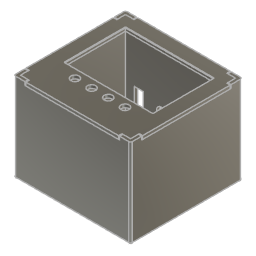
schnorriMat V1 (Autodesk Fusion 360 design; units mm, degrees)
Autodesk Fusion 360 part; units mm, degrees
sketch "Sketch2" plane through (0, 0, 0) normal (0, 0, 1) x (1, 0, 0)
  line L0 (-55, 60) -> (55, 60)
  line L1 (55, 60) -> (55, -60)
  line L2 (55, -60) -> (-55, -60)
  line L3 (-55, -60) -> (-55, 60)
  line L4 (0, 60) -> (0, -60) construction
  line L5 (55, 0) -> (-55, 0) construction
  line L6 (-55, 17.8) -> (55, 17.8) construction
  line L7 (-39.5, 45) -> (39.5, 45)
  line L8 (39.5, 45) -> (39.5, -9.4)
  line L9 (39.5, -9.4) -> (-39.5, -9.4)
  line L10 (-39.5, -9.4) -> (-39.5, 45)
  line L11 (39.5, 17.8) -> (-39.5, 17.8) construction
  line L12 (0, 45) -> (0, -9.4) construction
  line L13 (-55, -32) -> (55, -32) construction
  circle A0 centre (22.5, -32) radius 12.5
  circle A1 centre (-22.5, -32) radius 6.25
  line L14 (-6.3, -15.8) -> (-38.7, -15.8)
  line L15 (-38.7, -15.8) -> (-38.7, -48.2)
  line L16 (-38.7, -48.2) -> (-6.3, -48.2)
  line L17 (-6.3, -48.2) -> (-6.3, -15.8)
  line L18 (-6.3, -15.8) -> (-38.7, -48.2) construction
  line L19 (-38.7, -15.8) -> (-6.3, -48.2) construction
  line L20 (-4.3, -13.8) -> (-40.7, -13.8)
  line L21 (-40.7, -13.8) -> (-40.7, -50.2)
  line L22 (-40.7, -50.2) -> (-4.3, -50.2)
  line L23 (-4.3, -50.2) -> (-4.3, -13.8)
  line L24 (-32.5, -48.2) -> (-32.5, -50.2)
  line L25 (-38.7, -42) -> (-40.7, -42)
  line L26 (-22.5, -32) -> (-22.5, -50.2) construction
  point P0 (0, 17.8)
  point P1 (-22.5, -32)
  dimension "d1" = 110
  dimension "d6" = 120
  dimension "d7" = 79
  dimension "d8" = 54.4
  dimension "d9" = 15
  dimension "d12" = 25
  dimension "d13" = 12.5
  dimension "d15" = 32.4
  dimension "d16" = 32.4
  dimension "d17" = 45
  dimension "d18" = 22.5
  dimension "d19" = 28
  dimension "d42" = 2
  dimension "d63" = 10
  dimension "d64" = 10
  constraint horizontal L0
  constraint vertical L1
  constraint horizontal L2
  constraint vertical L3
  constraint midpoint L0 L4.start
  constraint midpoint L2 L4.end
  constraint midpoint L1 L5.start
  constraint midpoint L3 L5.end
  constraint midpoint L4 origin
  constraint coincident L3 L6.start
  constraint coincident L1 L6.end
  constraint perpendicular L1 L6
  constraint horizontal L7
  constraint vertical L8
  constraint horizontal L9
  constraint vertical L10
  constraint midpoint L8 L11.start
  constraint midpoint L10 L11.end
  constraint midpoint L7 L12.start
  constraint midpoint L9 L12.end
  constraint midpoint L11 P0
  constraint coincident L4 P0
  constraint collinear L6 L11
  constraint coincident L3 L13.start
  constraint coincident L1 L13.end
  constraint perpendicular L1 L13
  constraint coincident L13 A0.centre
  constraint coincident L13 P1
  constraint horizontal L14
  constraint perpendicular L14 L15
  constraint parallel L14 L16
  constraint parallel L15 L17
  constraint coincident L18 P1
  constraint coincident L19 P1
  constraint coincident P1 A1.centre
  constraint coincident L16 L24.start
  constraint perpendicular L16 L24
  constraint coincident L22 L24.end
  constraint coincident L15 L25.start
  constraint coincident L21 L25.end
  constraint perpendicular L21 L25
  constraint midpoint L22 L26.end
  measures "d1" distance of L0.start L0.end
  measures "d6" distance of L0.start L2.end
  measures "d7" distance of L7.start L7.end
  measures "d8" distance of L7.end L8.end
  measures "d9" distance of L0 L7
  measures "d12" diameter of A0
  measures "d13" diameter of A1
  measures "d15" distance of L15.end L16.end
  measures "d16" distance of L14.end L15.end
  measures "d17" distance of A0.centre P1
  measures "d18" distance of L4 P1
  measures "d19" distance of L2 L13
  measures "d63" distance of L13 L25
  measures "d64" distance of L24 L26
sketch "Sketch3" plane through (0, 0, 0) normal (0, 0, 1) x (1, 0, 0)
  line L0 (-55, 60) -> (55, 60)
  line L1 (55, 60) -> (55, -60)
  line L2 (55, -60) -> (-55, -60)
  line L3 (-55, -60) -> (-55, 60)
  line L4 (55, 0) -> (-55, 0) construction
  line L5 (0, 60) -> (0, -60) construction
  line L6 (-52.6, 57.6) -> (52.6, 57.6)
  line L7 (52.6, 57.6) -> (52.6, -57.6)
  line L8 (52.6, -57.6) -> (-52.6, -57.6)
  line L9 (-52.6, -57.6) -> (-52.6, 57.6)
  line L10 (-39.6, 57.6) -> (-39.6, 44.6)
  line L11 (-39.6, 44.6) -> (-52.6, 44.6)
  line L12 (-39.6, 51.1) -> (-52.6, 51.1) construction
  line L13 (-46.1, 44.6) -> (-46.1, 57.6) construction
  circle A0 centre (-46.1, 51.1) radius 5
  line L14 (-40.4, 57.6) -> (-40.4, 60)
  line L15 (-52.6, 45.4) -> (-55, 45.4)
  line L16 (-52.6, 44.6) -> (-55, 44.6)
  line L17 (-39.6, 57.6) -> (-39.6, 60)
  line L18 (39.6, 57.6) -> (39.6, 60)
  line L19 (40.4, 57.6) -> (40.4, 60)
  circle A1 centre (46.1, 51.1) radius 5
  line L20 (39.6, 57.6) -> (39.6, 44.6)
  line L21 (39.6, 44.6) -> (52.6, 44.6)
  line L22 (52.6, 44.6) -> (55, 44.6)
  line L23 (52.6, 45.4) -> (55, 45.4)
  line L24 (40.4, -57.6) -> (40.4, -60)
  line L25 (39.6, -57.6) -> (39.6, -60)
  line L26 (39.6, -57.6) -> (39.6, -44.6)
  circle A2 centre (46.1, -51.1) radius 5
  line L27 (39.6, -44.6) -> (52.6, -44.6)
  line L28 (52.6, -44.6) -> (55, -44.6)
  line L29 (52.6, -45.4) -> (55, -45.4)
  line L30 (-39.6, -57.6) -> (-39.6, -44.6)
  line L31 (-39.6, -57.6) -> (-39.6, -60)
  line L32 (-40.4, -57.6) -> (-40.4, -60)
  circle A3 centre (-46.1, -51.1) radius 5
  line L33 (-39.6, -44.6) -> (-52.6, -44.6)
  line L34 (-52.6, -44.6) -> (-55, -44.6)
  line L35 (-52.6, -45.4) -> (-55, -45.4)
  dimension "d20" = 110
  dimension "d21" = 120
  dimension "d22" = 2.4
  dimension "d23" = 13
  dimension "d26" = 10
  dimension "d27" = 0.8
  dimension "d28" = 0.8
  constraint horizontal L0
  constraint vertical L1
  constraint horizontal L2
  constraint vertical L3
  constraint midpoint L1 L4.start
  constraint midpoint L3 L4.end
  constraint midpoint L0 L5.start
  constraint midpoint L2 L5.end
  constraint midpoint L4 origin
  constraint coincident L6 L10.start
  constraint perpendicular L6 L10
  constraint coincident L9 L11.end
  constraint perpendicular L9 L11
  constraint midpoint L10 L12.start
  constraint coincident L9 L12.end
  constraint perpendicular L9 L12
  constraint midpoint L11 L13.start
  constraint coincident L6 L13.end
  constraint perpendicular L6 L13
  constraint midpoint L12 A0.centre
  constraint equal L10 L11
  constraint coincident L6 L14.start
  constraint coincident L0 L14.end
  constraint perpendicular L0 L14
  constraint coincident L9 L15.start
  constraint coincident L3 L15.end
  constraint perpendicular L3 L15
  constraint coincident L3 L16.end
  constraint perpendicular L3 L16
  constraint coincident L0 L17.end
  constraint perpendicular L0 L17
  constraint symmetric L5 L10.start L18.start
  constraint symmetric L5 L10.end L20.end
  constraint symmetric L5 L11.end L21.end
  constraint symmetric L5 A0 A1
  constraint symmetric L5 L14.start L19.start
  constraint symmetric L5 L14.end L19.end
  constraint symmetric L5 L15.start L23.start
  constraint symmetric L5 L15.end L23.end
  constraint symmetric L5 L16.end L22.end
  constraint symmetric L5 L17.end L18.end
  constraint symmetric L4 L10.start L30.start
  constraint symmetric L4 L10.end L30.end
  constraint symmetric L4 L11.end L33.end
  constraint symmetric L4 A0 A3
  constraint symmetric L4 L14.start L32.start
  constraint symmetric L4 L14.end L32.end
  constraint symmetric L4 L15.start L35.start
  constraint symmetric L4 L15.end L35.end
  constraint symmetric L4 L16.end L34.end
  constraint symmetric L4 L17.end L31.end
  constraint symmetric L4 L18.start L25.start
  constraint symmetric L4 L18.end L25.end
  constraint symmetric L4 L19.start L24.start
  constraint symmetric L4 L19.end L24.end
  constraint symmetric L4 A1 A2
  constraint symmetric L4 L20.end L26.end
  constraint symmetric L4 L21.end L27.end
  constraint symmetric L4 L22.end L28.end
  constraint symmetric L4 L23.start L29.start
  constraint symmetric L4 L23.end L29.end
  measures "d20" distance of L0.start L0.end
  measures "d21" distance of L0.start L2.end
  measures "d23" distance of L10.start L10.end
  measures "d26" diameter of A0
  measures "d27" distance of L14 L17
  measures "d28" distance of L15 L16
extrude "Extrude1" add sketch "Sketch3" along normal blind 2 contours L0 L3 L6 L9 L14 L15 | L0 L6 L14 L17 | L3 L9 L15 L16 | L0 L6 L17 L18 | L6 L9 L10 L11 | L3 L9 L16 L34 | L0 L6 L18 L19 | L6 L7 L8 L9 L10 L11 L20 L21 L26 L27 L30 L33 | L3 L9 L34 L35 | L0 L1 L6 L7 L19 L23 | L6 L7 L20 L21 | L2 L3 L8 L9 L32 L35 | L8 L9 L30 L33 | L1 L7 L22 L23 | L1 L7 L22 L28 | L2 L8 L31 L32 | L2 L8 L25 L31 | L1 L7 L28 L29 | L7 L8 L26 L27 | L2 L8 L24 L25 | L1 L2 L7 L8 L24 L29 | A0 | A1 | A2 | A3 makes body 1
extrude "Extrude2" add sketch "Sketch3" along normal blind 77 contours L0 L3 L6 L9 L14 L15 | L0 L6 L14 L17 | L3 L9 L15 L16 | L0 L6 L17 L18 | L3 L9 L16 L34 | L0 L6 L18 L19 | L3 L9 L34 L35 | L0 L1 L6 L7 L19 L23 | L2 L3 L8 L9 L32 L35 | L1 L7 L22 L23 | L1 L7 L22 L28 | L2 L8 L31 L32 | L2 L8 L25 L31 | L1 L7 L28 L29 | L2 L8 L24 L25 | L1 L2 L7 L8 L24 L29 bodies 1
extrude "Extrude3" add sketch "Sketch3" along normal blind 3 from surface at 77 contours L0 L3 L6 L9 L14 L15 | L0 L1 L6 L7 L19 L23 | L2 L3 L8 L9 L32 L35 | L1 L2 L7 L8 L24 L29 bodies 1
extrude "Extrude4" add sketch "Sketch2" along normal blind 3 from surface at 77 separate body contours L0 L1 L2 L3 | L14 L15 L16 L17 | L14 L15 L16 L17 L20 L21 L22 L23 L24 L25 | L15 L16 L21 L22 L24 L25 makes body 2
extrude "Extrude5" cut sketch "Sketch3" along normal through all contours L0 L3 L6 L9 L14 L15 | L0 L6 L14 L17 | L3 L9 L15 L16 | L0 L6 L18 L19 | L3 L9 L34 L35 | L0 L1 L6 L7 L19 L23 | L2 L3 L8 L9 L32 L35 | L1 L7 L22 L23 | L2 L8 L31 L32 | L1 L7 L28 L29 | L2 L8 L24 L25 | L1 L2 L7 L8 L24 L29 bodies 2
extrude "Extrude6" add sketch "Sketch3" along normal up to surface (75 mm away) from surface at 2 contours L6 L9 L10 L11 | L6 L7 L20 L21 | L8 L9 L30 L33 | L7 L8 L26 L27 | A0 | A1 | A2 | A3 bodies 1
extrude "Extrude7" cut sketch "Sketch3" against normal blind 1.5 from surface at 77 contours A0 | A1 | A2 | A3 bodies 1
fillet "Fillet1" radius 0.4 4 edges at (-52.6, 57.6, 78.5) (52.6, 57.6, 78.5) (52.6, -57.6, 78.5) (-52.6, -57.6, 78.5) on bodies 2
extrude "Extrude8" add sketch "Sketch2" against normal blind 5 from surface at 77 contours L14 L15 L16 L17 L20 L21 L22 L23 L24 L25 bodies 2
extrude "Extrude9" cut sketch "Sketch3" along normal blind 1.5 from surface at 77 contours A0 | A1 | A2 | A3 bodies 2
fillet "Fillet2" radius 5 4 edges at (-39.6, -44.6, 39.5) (-39.6, 44.6, 39.5) (39.6, 44.6, 39.5) (39.6, -44.6, 39.5) on bodies 1
fillet "Fillet4" radius 2.5 8 edges at (39.6, 57.6, 39.5) (52.6, 44.6, 39.5) (52.6, -44.6, 39.5) (39.6, -57.6, 39.5) (-39.6, -57.6, 39.5) (-52.6, -44.6, 39.5) (-52.6, 44.6, 39.5) (-39.6, 57.6, 39.5) on bodies 1
fillet "Fillet5" radius 1.2 4 edges at (55, 60, 40) (-55, 60, 40) (-55, -60, 40) (55, -60, 40) on bodies 1
sketch "Sketch5" plane through (0, 0, 0) normal (0, 1, 0) x (1, 0, 0)
  line L0 (-55, 0) -> (55, 0)
  line L1 (55, 0) -> (55, -80)
  line L2 (55, -80) -> (-55, -80)
  line L3 (-55, -80) -> (-55, 0)
  line L4 (55, -20) -> (-55, -20) construction
  circle A0 centre (-35, -20) radius 4
  line L5 (-19, -28) -> (-11, -28)
  line L6 (-11, -28) -> (-11, -12)
  line L7 (-11, -12) -> (-19, -12)
  line L8 (-19, -12) -> (-19, -28)
  line L9 (-19, -20) -> (-11, -20) construction
  line L10 (-15, -28) -> (-15, -12) construction
  dimension "d69" = 80
  dimension "d70" = 110
  dimension "d71" = 8
  dimension "d72" = 8
  dimension "d73" = 16
  dimension "d74" = 20
  dimension "d75" = 20
  dimension "d76" = 20
  constraint horizontal L0
  constraint vertical L1
  constraint horizontal L2
  constraint vertical L3
  constraint midpoint L0 origin
  constraint coincident L1 L4.start
  constraint coincident L3 L4.end
  constraint perpendicular L3 L4
  constraint coincident L4 A0.centre
  constraint horizontal L5
  constraint vertical L6
  constraint horizontal L7
  constraint vertical L8
  constraint midpoint L8 L9.start
  constraint midpoint L6 L9.end
  constraint midpoint L5 L10.start
  constraint midpoint L7 L10.end
  constraint collinear L4 L9
  measures "d69" distance of L0.start L2.end
  measures "d70" distance of L0.start L0.end
  measures "d71" diameter of A0
  measures "d72" distance of L5.start L5.end
  measures "d73" distance of L5.start L7.end
  measures "d74" distance of A0.centre L10
  measures "d75" distance of L0 L4
  measures "d76" distance of L3 A0.centre
extrude "Extrude10" cut sketch "Sketch5" along normal blind 85 contours A0 | L5 L6 L7 L8 bodies 1
sketch "Sketch1" plane through (0, 0, 0) normal (0, 0, 1) x (1, 0, 0) in component "V2"
  line L0 (39.5, 27.2) -> (-39.5, 27.2)
  line L1 (-39.5, 27.2) -> (-39.5, -27.2)
  line L2 (-39.5, -27.2) -> (39.5, -27.2)
  line L3 (39.5, -27.2) -> (39.5, 27.2)
  line L4 (39.5, 27.2) -> (-39.5, -27.2) construction
  line L5 (-39.5, 27.2) -> (39.5, -27.2) construction
  line L6 (-49.5, 37.2) -> (49.5, 37.2)
  line L7 (49.5, 37.2) -> (49.5, -57.2)
  line L8 (49.5, -57.2) -> (-49.5, -57.2)
  line L9 (-49.5, -57.2) -> (-49.5, 37.2)
  line L10 (0, 37.2) -> (0, -57.2) construction
  line L11 (-49.5, -35.2) -> (49.5, -35.2) construction
  circle A0 centre (-7.5, -35.2) radius 3.7
  circle A1 centre (-22.5, -35.2) radius 3.7
  circle A2 centre (22.5, -35.2) radius 3.7
  circle A3 centre (7.5, -35.2) radius 3.7
  line L12 (52.5, 40.2) -> (52.5, -60.2)
  line L13 (52.5, -60.2) -> (-52.5, -60.2)
  line L14 (-52.5, -60.2) -> (-52.5, 40.2)
  line L15 (-52.5, 40.2) -> (52.5, 40.2)
  dimension "d79" = 79
  dimension "d80" = 54.4
  dimension "d81" = 10
  dimension "d82" = 10
  dimension "d83" = 30
  dimension "d85" = 7.4
  dimension "d86" = 15
  dimension "d87" = 7.5
  dimension "d88" = -3
  dimension "d109" = 8
  constraint horizontal L0
  constraint perpendicular L0 L1
  constraint parallel L0 L2
  constraint parallel L1 L3
  constraint coincident L4 origin
  constraint coincident L5 origin
  constraint horizontal L6
  constraint vertical L7
  constraint horizontal L8
  constraint vertical L9
  constraint midpoint L6 L10.start
  constraint midpoint L8 L10.end
  constraint coincident origin L10
  constraint coincident L9 L11.start
  constraint coincident L7 L11.end
  constraint perpendicular L7 L11
  constraint coincident L11 A0.centre
  constraint coincident L11 A1.centre
  constraint equal A0 A1
  constraint symmetric L10 A0 A3
  constraint symmetric L10 A1 A2
  measures "d79" distance of L1.end L2.end
  measures "d80" distance of L0.end L1.end
  measures "d81" distance of L0 L6
  measures "d82" distance of L1 L9
  measures "d83" distance of L2 L8
  measures "d85" diameter of A0
  measures "d86" distance of A0.centre A1.centre
  measures "d87" distance of L10 A0.centre
  measures "d109" distance of L2 L11
sketch "Sketch2 (2)" plane through (0, 0, 0) normal (0, 0, 1) x (1, 0, 0) in component "V2"
  line L0 (-49.5, 37.2) -> (49.5, 37.2)
  line L1 (49.5, 37.2) -> (49.5, -57.2)
  line L2 (49.5, -57.2) -> (-49.5, -57.2)
  line L3 (-49.5, -57.2) -> (-49.5, 37.2)
  line L4 (-52.5, 40.2) -> (52.5, 40.2)
  line L5 (52.5, 40.2) -> (52.5, -60.2)
  line L6 (52.5, -60.2) -> (-52.5, -60.2)
  line L7 (-52.5, -60.2) -> (-52.5, 40.2)
  line L8 (0, 40.2) -> (0, -60.2) construction
  line L9 (52.5, -10) -> (-52.5, -10) construction
  line L10 (-42.5, 40.2) -> (-42.5, 37.2)
  line L11 (-41.7, 40.2) -> (-41.7, 37.2)
  line L12 (-49.5, 30.2) -> (-52.5, 30.2)
  line L13 (-52.5, 29.4) -> (-49.5, 29.4)
  line L14 (41.7, 40.2) -> (41.7, 37.2)
  line L15 (42.5, 40.2) -> (42.5, 37.2)
  line L16 (49.5, 30.2) -> (52.5, 30.2)
  line L17 (52.5, 29.4) -> (49.5, 29.4)
  line L18 (-41.7, -60.2) -> (-41.7, -57.2)
  line L19 (-42.5, -60.2) -> (-42.5, -57.2)
  line L20 (-49.5, -50.2) -> (-52.5, -50.2)
  line L21 (-52.5, -49.4) -> (-49.5, -49.4)
  line L22 (42.5, -60.2) -> (42.5, -57.2)
  line L23 (41.7, -60.2) -> (41.7, -57.2)
  line L24 (49.5, -50.2) -> (52.5, -50.2)
  line L25 (52.5, -49.4) -> (49.5, -49.4)
  point P0 (-49.5, 37.2)
  point P1 (49.5, -57.2)
  dimension "d89" = -3
  dimension "d90" = 0.8
  dimension "d91" = 0.8
  dimension "d92" = 10
  dimension "d93" = 10
  constraint horizontal L0
  constraint vertical L1
  constraint horizontal L2
  constraint vertical L3
  constraint coincident P0 L0.start
  constraint coincident P1 L1.end
  constraint midpoint L4 L8.start
  constraint midpoint L6 L8.end
  constraint midpoint L5 L9.start
  constraint midpoint L7 L9.end
  constraint coincident L4 L10.start
  constraint coincident L0 L10.end
  constraint perpendicular L0 L10
  constraint coincident L4 L11.start
  constraint coincident L0 L11.end
  constraint perpendicular L0 L11
  constraint coincident L3 L12.start
  constraint coincident L7 L12.end
  constraint perpendicular L7 L12
  constraint coincident L7 L13.start
  constraint coincident L3 L13.end
  constraint perpendicular L3 L13
  constraint symmetric L8 L10.start L15.start
  constraint symmetric L8 L10.end L15.end
  constraint symmetric L8 L11.start L14.start
  constraint symmetric L8 L11.end L14.end
  constraint symmetric L8 L12.start L16.start
  constraint symmetric L8 L12.end L16.end
  constraint symmetric L8 L13.start L17.start
  constraint symmetric L8 L13.end L17.end
  constraint symmetric L9 L10.start L19.start
  constraint symmetric L9 L10.end L19.end
  constraint symmetric L9 L11.start L18.start
  constraint symmetric L9 L11.end L18.end
  constraint symmetric L9 L12.start L20.start
  constraint symmetric L9 L12.end L20.end
  constraint symmetric L9 L13.start L21.start
  constraint symmetric L9 L13.end L21.end
  constraint symmetric L9 L14.start L23.start
  constraint symmetric L9 L14.end L23.end
  constraint symmetric L9 L15.start L22.start
  constraint symmetric L9 L15.end L22.end
  constraint symmetric L9 L16.start L24.start
  constraint symmetric L9 L16.end L24.end
  constraint symmetric L9 L17.start L25.start
  constraint symmetric L9 L17.end L25.end
  measures "d90" distance of L10 L11
  measures "d91" distance of L12 L13
  measures "d92" distance of L7 L10
  measures "d93" distance of L4 L12
extrude "Extrude2'" add sketch "Sketch2 (2)" along normal blind 2 separate body makes body 3 in component "V2"
extrude "Extrude3'" add sketch "Sketch2 (2)" along normal blind 77 contours L0 L3 L4 L7 L10 L12 | L0 L4 L10 L11 | L3 L7 L12 L13 | L0 L4 L11 L14 | L3 L7 L13 L21 | L0 L4 L14 L15 | L3 L7 L20 L21 | L0 L1 L4 L5 L15 L16 | L2 L3 L6 L7 L19 L20 | L1 L5 L16 L17 | L2 L6 L18 L19 | L1 L5 L17 L25 | L2 L6 L18 L23 | L1 L5 L24 L25 | L2 L6 L22 L23 | L1 L2 L5 L6 L22 L24 bodies 3 in component "V2"
extrude "Extrude4'" add sketch "Sketch2 (2)" along normal blind 3 from surface at 77 contours L0 L3 L4 L7 L10 L12 | L0 L1 L4 L5 L15 L16 | L2 L3 L6 L7 L19 L20 | L1 L2 L5 L6 L22 L24 bodies 3 in component "V2"
extrude "Extrude5'" add sketch "Sketch1" along normal blind 3 from surface at 77 separate body contours L6 L7 L8 L9 makes body 4 in component "V2"
extrude "Extrude6'" add sketch "Sketch2 (2)" along normal up to surface (3 mm away) from surface at 77 contours L0 L4 L11 L14 | L3 L7 L13 L21 | L1 L5 L17 L25 | L2 L6 L18 L23 bodies 4 in component "V2"
fillet "Fillet1'" radius 1.6 4 edges at (-52.5, -60.2, 40) (52.5, -60.2, 40) (52.5, 40.2, 40) (-52.5, 40.2, 40) on bodies 3 in component "V2"
fillet "Fillet2'" radius 1.4 8 edges at (52.0314, 39.7314, 0) (52.5, -10, 0) (52.0314, -59.7314, 0) (0, -60.2, 0) (-52.0314, -59.7314, 0) (-52.5, -10, 0) (-52.0314, 39.7314, 0) (0, 40.2, 0) on bodies 3 in component "V2"
fillet "Fillet3" radius 0.4 4 edges at (0, 27.2, 80) (39.5, 0, 80) (-39.5, 0, 80) (0, -27.2, 80) on bodies 4 in component "V2"
sketch "Sketch3 (2)" plane through (0, 0, 0) normal (0, 1, 0) x (1, 0, 0) in component "V2"
  line L0 (52.5, 0) -> (-52.5, 0)
  line L1 (-52.5, 0) -> (-52.5, -77)
  line L2 (-52.5, -77) -> (52.5, -77)
  line L3 (52.5, -77) -> (52.5, 0)
  line L4 (0, -77) -> (0, 0) construction
  line L5 (-52.5, -20) -> (52.5, -20) construction
  line L6 (-33.5, -28) -> (-41.5, -28)
  line L7 (-41.5, -28) -> (-41.5, -12)
  line L8 (-41.5, -12) -> (-33.5, -12)
  line L9 (-33.5, -12) -> (-33.5, -28)
  line L10 (-33.5, -20) -> (-41.5, -20) construction
  circle A0 centre (-17.5, -20) radius 4
  line L11 (-37.5, -28) -> (-37.5, -12) construction
  point P0 (52.5, 0)
  point P1 (-37.5, -20)
  dimension "d118" = 8
  dimension "d119" = 16
  dimension "d120" = 8
  dimension "d121" = 20
  dimension "d122" = 15
  dimension "d123" = 20
  constraint horizontal L0
  constraint vertical L1
  constraint horizontal L2
  constraint vertical L3
  constraint midpoint L2 L4.start
  constraint midpoint L0 L4.end
  constraint coincident L4.end origin
  constraint coincident P0 L0.start
  constraint coincident L1 L5.start
  constraint coincident L3 L5.end
  constraint perpendicular L3 L5
  constraint horizontal L6
  constraint vertical L7
  constraint horizontal L8
  constraint vertical L9
  constraint midpoint L9 L10.start
  constraint midpoint L7 L10.end
  constraint coincident L5 A0.centre
  constraint midpoint L6 L11.start
  constraint midpoint L8 L11.end
  constraint midpoint L11 P1
  constraint coincident L5 P1
  measures "d118" distance of L6.start L6.end
  measures "d119" distance of L6.start L8.end
  measures "d120" diameter of A0
  measures "d121" distance of L0 L5
  measures "d122" distance of L1 L11
  measures "d123" distance of A0.centre L11
extrude "Extrude7'" cut sketch "Sketch3 (2)" along normal blind 75 contours L6 L7 L8 L9 | A0 bodies 3 in component "V2"
delete_body "RemoveBody1" bodies 1
delete_body "RemoveBody2" bodies 2
component "V2" placed x (1, 0, 0) y (0, 1, 0) z (0, 0, 1) at (0, 0, 0)
equation "d1 = breiteTotal"
equation "breiteTotal = 110 mm"
equation "längeTotal = 120 mm"
equation "breiteDrucker = 79 mm" comment "gmessen 77.5"
equation "längeDrucker = 54.4 mm" comment "gem: 53.8"
equation "d6 = längeTotal"
equation "d7 = breiteDrucker"
equation "d8 = längeDrucker"
equation "buttonLoch = 25 mm"
equation "modusSwitch = 12.5 mm"
equation "d12 = buttonLoch"
equation "d13 = modusSwitch"
equation "modusSwitchPlatte = 32.4 mm"
equation "d15 = modusSwitchPlatte"
equation "d16 = modusSwitchPlatte"
equation "d18 = d17 / 2"
equation "d20 = breiteTotal"
equation "d21 = längeTotal"
equation "magnetDurchmesser = 10 mm"
equation "deckelDicke = 3 mm"
equation "gesamtHöhe = 80 mm"
equation "d33 = gesamtHöhe - deckelDicke"
equation "d36 = deckelDicke"
equation "d38 = deckelDicke"
equation "magnetDicke = 1.5 mm"
equation "d48 = -magnetDicke"
equation "d57 = magnetDicke"
equation "d69 = gesamtHöhe"
equation "d70 = breiteTotal"
equation "d79 = breiteDrucker"
equation "d80 = längeDrucker"
equation "smallButtonDurchmesser = 7.4 mm"
equation "d85 = smallButtonDurchmesser"
equation "d87 = d86 / 2"
equation "d98 = gesamtHöhe - deckelDicke"
equation "d101 = deckelDicke"
equation "d104 = deckelDicke"
named bodies: "Body", "Deckel", "schnorrimat_Box_V2", "schnorrimat_Deckel_V2"
